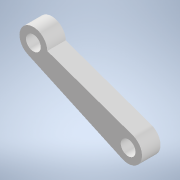
# Autodesk Inventor part: Palanca metacarpo_distal
Saved by Autodesk Inventor 2020 (Build 240168000, 168)
## iProperties
Created: 2021-08-20
Part Number: Palanca metacarpo_distal
Material: Generic
Document SubType Name: Modeling
Designer: chalo
Density: 1 g/cm^3
Appearance: Default
Author: chalo
Autodesk Inventor part; units mm, degrees
ref_plane "YZ Plane" through (0, 0, 0) normal (1, 0, 0) x (0, 1, 0)
ref_plane "XZ Plane" through (0, 0, 0) normal (0, 1, 0) x (-1, 0, 0)
ref_plane "XY Plane" through (0, 0, 0) normal (0, 0, 1) x (1, 0, 0)
sketch "Sketch1" plane through (0, 0, 0) normal (0, 0, 1) x (1, 0, 0)
  circle A0 centre (91.35, 6.3991) radius 1.6 projected
  circle A1 centre (70.85, 15.7754) radius 1.6 projected
  circle A2 centre (70.85, 15.7754) radius 3
  circle A3 centre (91.35, 6.3991) radius 3
  line L0 (69.6022, 13.0472) -> (90.1022, 3.671)
  line L1 (73.85, 15.7754) -> (92.351, 9.2272)
  point P0 (0, 0)
  dimension "d0" = 6
  dimension "d1" = 6
  constraints: 4 end point, 4 point on circle, 3 tangent, 2 centre point, 2 coincident, 1 horizontal alignment
  measures "d0" diameter of A2
  measures "d1" diameter of A3
extrude "Extrusion1" add sketch "Sketch1" along normal mid plane 4
body "Solid1"
